Autodesk Fusion 360 part; units mm, degrees
(part 3 of 3)
sketch "Schizzo38" plane through (-271.3139, 0, 0) normal (-1, 0, 0) x (0, -1, 0)
  line L0 (10.9044, 16) -> (30.9044, 16)
  line L1 (30.9044, 16) -> (30.9044, 140)
  line L2 (19.4044, 140) -> (10.9044, 140)
  line L3 (10.9044, 140) -> (10.9044, 16)
  line L4 (19.4044, 140) -> (10.9044, 140) construction
  line L5 (10.9044, 140) -> (10.9044, 123.5) construction
  line L6 (10.9044, 123.5) -> (19.4044, 123.5) construction
  line L7 (19.4044, 123.5) -> (19.4044, 140) construction
  line L8 (28.9044, 123.5) -> (24.9044, 123.5)
  line L9 (24.9044, 123.5) -> (24.9044, 140)
  line L10 (24.9044, 140) -> (28.9044, 140)
  line L11 (28.9044, 140) -> (28.9044, 123.5)
  line L12 (26.9044, 123.5) -> (26.9044, 140) construction
  line L13 (19.4044, 123.5) -> (19.4044, 140)
  line L14 (30.9044, 140) -> (22.4044, 140)
  line L15 (22.4044, 140) -> (22.4044, 123.5)
  line L16 (22.4044, 123.5) -> (19.4044, 123.5)
  point P0 (10.9044, 140)
  dimension "d411" = 16.5
  dimension "d412" = 4
  dimension "d419" = 4
  constraint horizontal L4
  constraint vertical L5
  constraint horizontal L6
  constraint vertical L7
  constraint coincident L2.start L4.start
  constraint coincident P0 L2.end
  constraint horizontal L8
  constraint vertical L9
  constraint horizontal L10
  constraint vertical L11
  constraint coincident L4 L9.end
  constraint coincident L6 L8.start
  constraint midpoint L8 L12.start
  constraint midpoint L10 L12.end
  measures "d411" distance of L4 L6
  measures "d412" distance of L9 L11
  measures "d419" distance of L1 L12
extrude "Estrusione95" cut sketch "Schizzo38" against normal blind 5 contours L8 L9 L10 L11 L14 bodies 9
sketch "Schizzo28" plane through (0, -30.9044, 0) normal (0, -1, 0) x (1, 0, 0)
  line L0 (-261.8139, 0) -> (-253.3139, 0)
  line L1 (-253.3139, 0) -> (-253.3139, 16)
  line L2 (-255.3139, 16) -> (-255.3139, 140)
  line L3 (-255.3139, 140) -> (-271.3139, 140)
  line L4 (-271.3139, 140) -> (-271.3139, 16)
  line L5 (-273.3139, 16) -> (-273.3139, 0)
  line L6 (-273.3139, 0) -> (-273.3139, 16) construction
  line L7 (-273.3139, 0) -> (-253.3139, 0) construction
  line L8 (-261.8139, 0) -> (-253.3139, 0)
  line L9 (-253.3139, 0) -> (-253.3139, 16.5)
  line L10 (-261.8139, 20.1122) -> (-261.8139, 0)
  line L11 (-263.3139, 0) -> (-263.3139, 16.5) construction
  line L12 (-263.3139, 140) -> (-263.3139, 15) construction
  line L13 (-271.3139, 132) -> (-255.3139, 132) construction
  circle A0 centre (-263.3139, 132) radius 8
  circle A1 centre (-263.3139, 132) radius 4.1
  circle A2 centre (-263.3139, 132) radius 2
  line L14 (-261.8139, 16.5) -> (-261.8139, 0)
  line L15 (-273.3139, 0) -> (-264.8139, 0)
  line L16 (-264.8139, 0) -> (-264.8139, 16.5)
  line L17 (-264.8139, 16.5) -> (-261.8139, 16.5)
  line L18 (-261.8139, 16.5) -> (-261.8139, 0)
  line L19 (-261.8139, 0) -> (-253.3139, 0)
  line L20 (-253.3139, 0) -> (-253.3139, 16)
  line L21 (-253.3139, 16) -> (-255.3139, 16)
  line L22 (-255.3139, 16) -> (-255.3139, 140)
  line L23 (-271.3139, 140) -> (-271.3139, 16)
  line L24 (-271.3139, 16) -> (-273.3139, 16)
  line L25 (-273.3139, 16) -> (-273.3139, 0)
  line L26 (-273.3139, 0) -> (-264.8139, 0)
  line L27 (-264.8139, 0) -> (-264.8139, 16.5)
  line L28 (-264.8139, 16.5) -> (-261.8139, 16.5)
  line L29 (-273.3139, 16.5) -> (-253.3139, 16.5)
  line L30 (-253.3139, 16.5) -> (-253.3139, 0)
  line L31 (-253.3139, 0) -> (-273.3139, 0)
  line L32 (-273.3139, 0) -> (-273.3139, 16.5)
  line L33 (-255.3139, 140) -> (-271.3139, 140)
  line L34 (-263.3139, 136.1) -> (-271.3139, 136.1)
  line L35 (-271.3139, 136.1) -> (-271.3139, 127.9)
  line L36 (-271.3139, 127.9) -> (-263.3139, 127.9)
  line L37 (-263.3139, 127.9) -> (-263.3139, 136.1)
  point P0 (-271.3139, 0)
  dimension "d343" = 8
  dimension "d344" = 8.2
  dimension "d345" = 4
  dimension "d355" = 16.5
  constraint coincident L0.end L1.start
  constraint perpendicular L1 L7
  constraint horizontal L8
  constraint vertical L9
  constraint vertical L10
  constraint coincident L0.start L8.start
  constraint coincident L0.end L9
  constraint midpoint L7 L11.start
  constraint midpoint L3 L12.start
  constraint coincident L11 L12.end
  constraint coincident L4 L13.start
  constraint coincident L2 L13.end
  constraint perpendicular L12 L13
  constraint midpoint L13 A0.centre
  constraint tangent L3 A0
  constraint concentric A0 A1
  constraint concentric A0 A2
  constraint horizontal L29
  constraint vertical L30
  constraint horizontal L31
  constraint vertical L32
  constraint coincident L5.end L6.start
  constraint horizontal L34
  constraint vertical L35
  constraint horizontal L36
  constraint vertical L37
  constraint coincident A1 L34.start
  constraint coincident L12 L34.start
  constraint tangent A0 L35
  constraint tangent A1 L36
  measures "d343" distance of L3 L13.start
  measures "d344" diameter of A1
  measures "d345" diameter of A2
  measures "d355" distance of L29 P0
extrude "Estrusione80" cut sketch "Schizzo28" against normal blind 20 contours A2 L37 | A2 L37 bodies 9
extrude "Estrusione79" cut sketch "Schizzo28" against normal blind 1.5 contours A1 A2 L37 | A1 A2 L37 bodies 9
extrude "Estrusione81" cut sketch "Schizzo28" along normal blind 1 from surface at -20 contours A1 A2 L37 | A1 A2 L37 bodies 9
extrude "Estrusione122" cut sketch "Schizzo28" along normal blind 0.5 from surface at -20 contours L4 A0 L23 L35 L36 | A0 A1 L34 L36 | L4 A0 L23 L34 L35 picked at (-269.986, 131.5402) bodies 9
extrude "Estrusione82" cut sketch "Schizzo28" against normal blind 20 contours L2 L3 A0 L22 L33 | L3 L4 A0 L23 L33 L34 | L4 A0 L23 L34 L35 bodies 9
extrude "Estrusione77" cut sketch "Schizzo28" against normal blind 2 contours L0 L1 L2 L8 L9 L10 L14 L18 L19 L20 L21 L22 L29 L30 L31 | L4 L5 L15 L16 L23 L24 L25 L26 L27 L29 L31 L32 bodies 9
extrude "Estrusione78" cut sketch "Schizzo28" along normal blind 2 from surface at -20 contours L0 L1 L2 L8 L9 L10 L14 L18 L19 L20 L21 L22 L29 L30 L31 | L4 L5 L15 L16 L23 L24 L25 L26 L27 L29 L31 L32 bodies 9
sketch "Schizzo27" plane through (-273.3139, 0, 0) normal (-1, 0, 0) x (0, -1, 0)
  line L0 (12.9044, 0) -> (28.9044, 0)
  line L1 (28.9044, 16) -> (12.9044, 16)
  line L2 (12.9044, 16) -> (28.9044, 16) construction
  line L3 (28.9044, 16) -> (28.9044, 0) construction
  line L4 (28.9044, 0) -> (12.9044, 0) construction
  line L5 (12.9044, 0) -> (12.9044, 16) construction
  line L6 (20.9044, 16) -> (20.9044, 0) construction
  line L7 (12.9044, 8) -> (28.9044, 8)
  circle A0 centre (20.9044, 8) radius 8
  circle A1 centre (20.9044, 8) radius 2
  circle A2 centre (20.9044, 8) radius 4.1
  line L8 (12.9044, 16) -> (12.9044, 0)
  line L9 (28.9044, 0) -> (28.9044, 16)
  line L10 (20.9044, 12.1) -> (12.9044, 12.1)
  line L11 (12.9044, 12.1) -> (12.9044, 3.9)
  line L12 (12.9044, 3.9) -> (20.9044, 3.9)
  line L13 (20.9044, 3.9) -> (20.9044, 12.1)
  dimension "d317" = 4
  dimension "d322" = 8.2
  constraint horizontal L2
  constraint vertical L3
  constraint horizontal L4
  constraint vertical L5
  constraint coincident L0.end L3.end
  constraint coincident L1.end L2.start
  constraint midpoint L2 L6.start
  constraint midpoint L4 L6.end
  constraint midpoint L5 L7.start
  constraint midpoint L3 L7.end
  constraint midpoint L6 A0.centre
  constraint tangent L4 A0
  constraint concentric A0 A1
  constraint concentric A1 A2
  constraint horizontal L10
  constraint vertical L11
  constraint horizontal L12
  constraint vertical L13
  constraint coincident A2 L10.start
  constraint coincident L6 L10.start
  constraint tangent A2 L12
  constraint tangent A0 L11
  measures "d317" diameter of A1
  measures "d322" diameter of A2
extrude "Estrusione71" cut sketch "Schizzo27" against normal blind 20 contours L7 A1 L13 | L7 A1 L13 | L7 A1 L13 | L7 A1 L13 bodies 9
extrude "Estrusione72" cut sketch "Schizzo27" against normal blind 2 contours L1 A0 L9 | A0 L8 L10 L11 | L1 A0 L8 L10 bodies 9
extrude "Estrusione73" cut sketch "Schizzo27" against normal blind 20 contours L0 A0 L8 L12 | L0 A0 L9 | A0 L8 L11 L12 bodies 9
extrude "Estrusione74" cut sketch "Schizzo27" against normal blind 2 from surface at -18 contours L1 A0 L9 | A0 L8 L10 L11 | L1 A0 L8 L10 bodies 9
extrude "Estrusione75" cut sketch "Schizzo27" against normal blind 1 contours L7 A1 A2 L13 | L7 A1 A2 L13 | L7 A1 A2 L13 | L7 A1 A2 L13 bodies 9
extrude "Estrusione123" cut sketch "Schizzo27" against normal blind 0.5 contours L7 A0 A2 L12 | L7 A0 A2 L10 picked at (14.919, 5.0184) picked at (14.919, 10.9816) bodies 9
extrude "Estrusione76" cut sketch "Schizzo27" along normal blind 1.5 from surface at -20 contours L7 A1 A2 L13 | L7 A1 A2 L13 | L7 A1 A2 L13 | L7 A1 A2 L13 bodies 9
extrude "Estrusione105" add sketch "Schizzo1" along normal blind 16 separate body contours L191 L192 L193 L194 | L195 L196 L198 L199 | L196 L197 L198 L199 | A21 | A21 L202 L203 L204 L212 L213 L216 L217 | A21 L201 L202 L204 L207 L208 L220 L223 | L201 L202 L207 L208 L209 L210 | L202 L203 L212 L213 L214 L215 | L203 L204 L216 L217 L218 L219 | L201 L204 L220 L221 L222 L223 | A22 makes body 10
sketch "Schizzo41" plane through (0, -6.7942, 0) normal (0, -1, 0) x (1, 0, 0)
  line L0 (-212.9415, 0) -> (-192.9415, 0)
  line L1 (-192.9415, 0) -> (-192.9415, 16)
  line L2 (-192.9415, 16) -> (-212.9415, 16)
  line L3 (-212.9415, 16) -> (-212.9415, 0)
  line L4 (-212.9415, 16) -> (-192.9415, 16) construction
  line L5 (-192.9415, 16) -> (-192.9415, 0) construction
  line L6 (-192.9415, 0) -> (-212.9415, 0) construction
  line L7 (-212.9415, 0) -> (-212.9415, 16) construction
  line L8 (-202.9415, 16) -> (-202.9415, 0) construction
  line L9 (-212.9415, 8) -> (-192.9415, 8) construction
  line L10 (-201.4415, 16) -> (-204.4415, 16)
  line L11 (-204.4415, 16) -> (-204.4415, 0)
  line L12 (-204.4415, 0) -> (-201.4415, 0)
  line L13 (-201.4415, 0) -> (-201.4415, 16)
  line L14 (-201.4415, 16) -> (-204.4415, 0) construction
  line L15 (-204.4415, 16) -> (-201.4415, 0) construction
  line L16 (-212.9415, 0) -> (-192.9415, 0) construction
  line L17 (-192.9415, 16) -> (-195.9415, 16) construction
  line L18 (-195.9415, 16) -> (-195.9415, 13) construction
  line L19 (-195.9415, 13) -> (-192.9415, 13) construction
  line L20 (-192.9415, 13) -> (-192.9415, 16) construction
  line L21 (-193.9415, 15) -> (-197.9415, 15)
  line L22 (-197.9415, 15) -> (-197.9415, 11)
  line L23 (-197.9415, 11) -> (-193.9415, 11)
  line L24 (-193.9415, 11) -> (-193.9415, 15)
  line L25 (-193.9415, 15) -> (-197.9415, 11) construction
  line L26 (-197.9415, 15) -> (-193.9415, 11) construction
  line L27 (-197.9415, 15) -> (-193.9415, 15)
  line L28 (-193.9415, 15) -> (-193.9415, 16)
  line L29 (-193.9415, 16) -> (-197.9415, 16)
  line L30 (-197.9415, 16) -> (-197.9415, 15)
  point P0 (-192.9415, 0)
  point P1 (-202.9415, 8)
  point P2 (-195.9415, 13)
  dimension "d463" = 3
  dimension "d464" = 3
  dimension "d465" = 3
  dimension "d466" = 4
  dimension "d467" = 4
  constraint horizontal L4
  constraint vertical L5
  constraint horizontal L6
  constraint vertical L7
  constraint coincident P0 L0.end
  constraint coincident L2.end L3.start
  constraint midpoint L4 L8.start
  constraint midpoint L6 L8.end
  constraint midpoint L7 L9.start
  constraint midpoint L5 L9.end
  constraint horizontal L10
  constraint perpendicular L10 L11
  constraint parallel L10 L12
  constraint parallel L11 L13
  constraint coincident L14 P1
  constraint coincident L15 P1
  constraint midpoint L9 P1
  constraint collinear L12 L16
  constraint horizontal L17
  constraint vertical L18
  constraint horizontal L19
  constraint vertical L20
  constraint coincident L1.end L2.start
  constraint horizontal L21
  constraint perpendicular L21 L22
  constraint parallel L21 L23
  constraint parallel L22 L24
  constraint coincident L25 P2
  constraint coincident L26 P2
  constraint coincident P2 L18.end
  constraint horizontal L27
  constraint vertical L28
  constraint horizontal L29
  constraint vertical L30
  constraint coincident L17 L28.end
  constraint coincident L21.start L24.end
  measures "d463" distance of L11.end L12.end
  measures "d464" distance of L1.end L17.end
  measures "d465" distance of L1.end L19.end
  measures "d466" distance of L22.end L23.end
  measures "d467" distance of L21.end L22.end
extrude "Estrusione106" cut sketch "Schizzo41" against normal blind 50 contours L21 L22 L23 L24 L27 bodies 10
extrude "Estrusione107" cut sketch "Schizzo41" against normal blind 16.5 contours L2 L21 L27 L28 L29 L30 bodies 10
extrude "Estrusione108" cut sketch "Schizzo41" against normal blind 16.5 contours L0 L2 L10 L11 L12 L13 bodies 10
extrude "Estrusione109" cut sketch "Schizzo1" against normal blind 6 from surface at 16 contours L195 L196 L198 L199 bodies 10
extrude "Estrusione110" cut sketch "Schizzo1" against normal blind 10 from surface at 16 contours L196 L197 L198 L199 bodies 10
extrude "Estrusione111" cut sketch "Schizzo1" along normal blind 16 contours A22 bodies 10
extrude "Estrusione112" cut sketch "Schizzo1" against normal blind 6.4 from surface at 16 contours A21 bodies 10
extrude "Estrusione113" cut sketch "Schizzo1" along normal blind 5 contours A21 | A21 L202 L203 L204 L212 L213 L216 L217 | A21 L201 L202 L204 L207 L208 L220 L223 | L201 L202 L207 L208 L209 L210 | L202 L203 L212 L213 L214 L215 | L203 L204 L216 L217 L218 L219 | L201 L204 L220 L221 L222 L223 bodies 10
extrude "Estrusione114" cut sketch "Schizzo1" along normal blind 10 contours L201 L202 L207 L208 L209 L210 | L202 L203 L212 L213 L214 L215 | L203 L204 L216 L217 L218 L219 | L201 L204 L220 L221 L222 L223 bodies 10
sketch "Schizzo42" plane through (-192.9415, 0, 0) normal (1, 0, 0) x (0, 1, 0)
  line L0 (-6.7942, 0) -> (133.2058, 0)
  line L1 (133.2058, 0) -> (133.2058, 16)
  line L2 (133.2058, 16) -> (-6.7942, 16)
  line L3 (-6.7942, 16) -> (-6.7942, 0)
sketch "Schizzo43" plane through (-192.9415, 0, 0) normal (1, 0, 0) x (0, 1, 0)
  line L0 (-6.7942, 16) -> (133.2058, 16)
  line L1 (133.2058, 16) -> (133.2058, 0) construction
  line L2 (133.2058, 0) -> (-6.7942, 0)
  line L3 (-6.7942, 0) -> (-6.7942, 16)
  line L4 (-6.7942, 8) -> (133.2058, 8) construction
  circle A0 centre (1.2058, 8) radius 8
  circle A1 centre (1.2058, 8) radius 2
  circle A2 centre (1.2058, 8) radius 4.1
  line L5 (-2.8942, 16) -> (5.3058, 16)
  line L6 (5.3058, 16) -> (5.3058, 0)
  line L7 (5.3058, 0) -> (-2.8942, 0)
  line L8 (-2.8942, 0) -> (-2.8942, 16)
  line L9 (-2.8942, 16) -> (5.3058, 0) construction
  line L10 (5.3058, 16) -> (-2.8942, 0) construction
  point P0 (133.2058, 0)
  point P1 (-6.7942, 16)
  point P2 (2.7058, 8)
  point P3 (1.2058, 8)
  dimension "d502" = 4
  dimension "d504" = 8.2
  constraint horizontal L0
  constraint vertical L1
  constraint horizontal L2
  constraint vertical L3
  constraint coincident P0 L1.end
  constraint coincident L0.start L3.end
  constraint midpoint L3 L4.start
  constraint midpoint L1 L4.end
  constraint coincident L4 P3
  constraint tangent L2 A0
  constraint tangent L3 A0
  constraint concentric A0 A1
  constraint concentric A1 A2
  constraint horizontal L5
  constraint perpendicular L5 L6
  constraint parallel L5 L7
  constraint parallel L6 L8
  constraint coincident L9 P3
  constraint coincident L10 P3
  constraint coincident P3 A0.centre
  constraint tangent A2 L6
  constraint tangent A0 L7
  measures "d502" diameter of A1
  measures "d504" diameter of A2
extrude "Estrusione115" cut sketch "Schizzo43" against normal blind 20 contours L0 L3 A0 L8 | L0 A0 L5 L8 | L2 L3 A0 L8 | L2 A0 L7 L8 bodies 10
extrude "Estrusione116" cut sketch "Schizzo43" against normal blind 20 contours A1 bodies 10
extrude "Estrusione117" cut sketch "Schizzo43" against normal blind 1 contours A2 bodies 10
extrude "Estrusione118" cut sketch "Schizzo43" along normal blind 1 from surface at -20 contours A2 bodies 10
extrude "Estrusione119" cut sketch "Schizzo43" along normal blind 0.5 from surface at -20 contours L0 A0 L5 L8 | L0 A0 L5 L6 | A0 A2 L6 L8 picked at (0.746, 14.6721) bodies 10
extrude "Estrusione125" add sketch "Schizzo1" along normal blind 1 separate body contours L224 L227 L230 L231 L234 L243 L266 L268 | L224 L229 A23 L230 L231 L234 L243 L246 | L227 L228 L230 L231 L234 L245 L265 L266 L267 | L224 L229 A24 L232 L234 L247 L249 | L230 L231 L234 L243 L246 | L230 L231 L234 L243 L244 L267 | L227 L228 L230 L231 L233 L235 L257 L258 L260 | L234 L244 L266 L267 L268 | L234 L244 L265 L266 L267 | L224 L225 L232 L234 L247 L271 L272 | L229 A24 L234 L253 | L229 A23 L234 L253 | L230 L231 L234 L245 L246 | L230 L231 L234 L244 L245 L267 | L226 L227 L230 L231 L233 L237 L259 L260 | L228 A23 L234 L252 L253 | A23 L230 L231 L234 L245 L246 | L228 A23 L233 L251 L252 | A23 L230 L231 L233 L235 L236 | L232 L234 L247 L248 L270 | L232 L234 L247 L249 | A23 L234 | L228 A24 L234 L253 L254 | A24 L234 | L233 L238 L257 L258 L260 | L233 L238 L258 L259 L260 | A23 L233 | L226 L229 A23 L230 L231 L233 L236 L237 | L230 L231 L233 L235 L236 | L230 L231 L233 L235 L238 L258 | L225 L228 L232 L234 L250 L269 L270 L271 | L232 L234 L248 L250 L270 | L232 L234 L249 L250 | L234 L248 L270 L271 L272 | A24 L232 L234 L249 L250 | L230 L231 L233 L237 L238 L258 | L229 A23 L233 L251 | L230 L231 L233 L236 L237 | L225 L228 L232 L233 L239 L261 L262 L263 | L234 L248 L269 L270 L271 | L229 A24 L233 L251 | L228 A24 L233 L251 L254 | A24 L232 L233 L239 L240 | L226 L229 A24 L232 L233 L240 L242 | L225 L226 L232 L233 L242 L261 L264 | A24 L233 | L232 L233 L239 L241 L262 | L232 L233 L239 L240 | L233 L241 L261 L262 L264 | L233 L241 L261 L262 L263 | L232 L233 L240 L242 | L232 L233 L241 L242 L262 makes body 11
extrude "Estrusione124" add sketch "Schizzo1" along normal blind 83 contours L224 L227 L230 L231 L234 L243 L266 L268 | L224 L229 A23 L230 L231 L234 L243 L246 | L227 L228 L230 L231 L234 L245 L265 L266 L267 | L224 L229 A24 L232 L234 L247 L249 | L227 L228 L230 L231 L233 L235 L257 L258 L260 | L224 L225 L232 L234 L247 L271 L272 | L226 L227 L230 L231 L233 L237 L259 L260 | A23 L230 L231 L234 L245 L246 | A23 L230 L231 L233 L235 L236 | A23 L234 | A24 L234 | A23 L233 | L226 L229 A23 L230 L231 L233 L236 L237 | L225 L228 L232 L234 L250 L269 L270 L271 | A24 L232 L234 L249 L250 | L225 L228 L232 L233 L239 L261 L262 L263 | A24 L232 L233 L239 L240 | L226 L229 A24 L232 L233 L240 L242 | L225 L226 L232 L233 L242 L261 L264 | A24 L233 bodies 11
sketch "Schizzo44" plane through (0, 21.6443, 0) normal (0, -1, 0) x (1, 0, 0)
  line L0 (-605.2788, 0) -> (-528.2788, 0)
  line L1 (-528.2788, 0) -> (-528.2788, 83)
  line L2 (-528.2788, 83) -> (-605.2788, 83)
  line L3 (-605.2788, 83) -> (-605.2788, 0)
  circle A0 centre (-566.7788, 41.75) radius 11
  line L4 (-605.2788, 83) -> (-528.2788, 83) construction
  line L5 (-528.2788, 83) -> (-528.2788, 0) construction
  line L6 (-528.2788, 0) -> (-605.2788, 0) construction
  line L7 (-605.2788, 0) -> (-605.2788, 83) construction
  line L8 (-566.7788, 0) -> (-566.7788, 83) construction
  dimension "d543" = 22
  dimension "d544" = 41.25
  dimension "d546" = 77
  dimension "d547" = 83
  constraint horizontal L4
  constraint vertical L5
  constraint horizontal L6
  constraint vertical L7
  constraint coincident L0.end L1.start
  constraint coincident L2.end L3.start
  constraint midpoint L6 L8.start
  constraint midpoint L4 L8.end
  constraint coincident A0.centre L8
  measures "d543" diameter of A0
  measures "d544" distance of A0.centre L4
  measures "d546" distance of L5 L7
  measures "d547" distance of L4 L6
extrude "Estrusione126" cut sketch "Schizzo44" against normal blind 2 contours A0 bodies 11
extrude "Estrusione129" add sketch "Schizzo1" along normal blind 2 separate body contours L291 L292 L293 L294 makes body 12
extrude "Estrusione130" add sketch "Schizzo1" along normal blind 10 contours L304 L305 L306 L307 L309 | L313 L316 L317 L318 | L322 L323 L324 L325 | L326 L327 L328 L329 bodies 12
extrude "Estrusione131" add sketch "Schizzo1" along normal blind 2 separate body contours L343 L344 L345 L346 | L347 L348 L350 L355 | L348 L349 L350 L355 L356 | L348 L349 L353 L354 L355 L356 L358 L360 L363 L364 L365 L367 A25 | L355 L357 L358 L359 | L354 L355 L357 L358 L360 | L353 L356 L361 L363 L364 | L353 L361 L362 L363 | L353 L354 L365 L367 L368 A25 | L353 L366 L367 L368 | L365 L367 A25 | L365 L367 A25 | A26 makes body 13
extrude "Estrusione132" add sketch "Schizzo1" along normal blind 55 contours L343 L344 L345 L346 bodies 13
extrude "Estrusione133" add sketch "Schizzo1" along normal blind 100 from surface at 30 contours L347 L348 L350 L355 | L348 L349 L350 L355 L356 | L355 L357 L358 L359 | L354 L355 L357 L358 L360 | L353 L356 L361 L363 L364 | L353 L361 L362 L363 | L353 L354 L365 L367 L368 A25 | L353 L366 L367 L368 | L365 L367 A25 picked at (-531.8187, -95.3723) bodies 13
sketch "Schizzo46" plane through (0, -106.2441, 0) normal (0, -1, 0) x (1, 0, 0)
  line L0 (-605.2788, 0) -> (-528.2788, 0)
  line L1 (-528.2788, 0) -> (-528.2788, 55)
  line L2 (-528.2788, 55) -> (-605.2788, 55)
  line L3 (-605.2788, 55) -> (-605.2788, 0)
  line L4 (-605.2788, 55) -> (-528.2788, 55) construction
  line L5 (-528.2788, 55) -> (-528.2788, 0) construction
  line L6 (-528.2788, 0) -> (-605.2788, 0) construction
  line L7 (-605.2788, 0) -> (-605.2788, 55) construction
  circle A0 centre (-542.2788, 8) radius 5.05
  line L8 (-605.2788, 0) -> (-528.2788, 0)
  line L9 (-542.2788, 8) -> (-542.2788, 55) construction
  line L10 (-538.0288, 27) -> (-546.5288, 27)
  line L11 (-546.5288, 27) -> (-546.5288, 41)
  line L12 (-546.5288, 41) -> (-538.0288, 41)
  line L13 (-538.0288, 41) -> (-538.0288, 27)
  line L14 (-538.0288, 27) -> (-546.5288, 41) construction
  line L15 (-546.5288, 27) -> (-538.0288, 41) construction
  line L16 (-605.2788, 27.5) -> (-528.2788, 27.5) construction
  line L17 (-542.2788, 13.05) -> (-528.2788, 13.05) construction
  point P0 (-528.2788, 0)
  point P1 (-542.2788, 34)
  dimension "d600" = 10.1
  dimension "d607" = 8
  dimension "d608" = 14
  dimension "d617" = 8.5
  dimension "d618" = 14
  dimension "d619" = 6.5
  dimension "d620" = 14
  dimension "d621" = 13.95
  constraint horizontal L4
  constraint vertical L5
  constraint horizontal L6
  constraint vertical L7
  constraint coincident L2.end L3.start
  constraint coincident P0 L0.end
  constraint coincident A0.centre L9.start
  constraint coincident L2 L9.end
  constraint perpendicular L2 L9
  constraint horizontal L10
  constraint perpendicular L10 L11
  constraint parallel L10 L12
  constraint parallel L11 L13
  constraint coincident L14 P1
  constraint coincident L15 P1
  constraint coincident L9 P1
  constraint midpoint L7 L16.start
  constraint midpoint L5 L16.end
  constraint coincident A0 L17.start
  constraint coincident L9 L17.start
  constraint coincident L5 L17.end
  constraint tangent A0 L17
  measures "d600" diameter of A0
  measures "d607" distance of L6 A0.centre
  measures "d608" distance of L5 A0.centre
  measures "d617" distance of L11.end L12.end
  measures "d618" distance of L10.end L11.end
  measures "d619" distance of P1 L16
  measures "d620" distance of L4 L12
  measures "d621" distance of L10 L17
extrude "Estrusione134" cut sketch "Schizzo46" against normal blind 3 contours A0 bodies 13
extrude "Estrusione135" cut sketch "Schizzo1" along normal blind 2 contours L365 L367 A25 | L365 L367 A25 | A26 bodies 13
extrude "Estrusione136" cut sketch "Schizzo46" against normal blind 2 contours L10 L11 L12 L13 bodies 13
equation "BeamLenght = 140 mm"
equation "d2 = BeamLenght"
equation "d4 = BeamLock"
equation "BeamSlotDepth = 16.5 mm"
equation "d10 = -BeamSlotDepth"
equation "d12 = -BeamSlotDepth"
equation "d68 = d67"
equation "d70 = d69"
equation "d73 = -4 mm - JointLockDepth"
equation "d75 = BeamScrewHole"
equation "d76 = JointLockDepth"
equation "d79 = -JointLockDepth"
equation "d89 = CableBoreSize"
equation "d90 = CableBoreSize"
equation "d93 = CableBoreSize"
equation "d94 = CableBoreSize"
equation "d129 = BeamSlotDepth"
equation "CableBoreSize = 4 mm"
equation "d132 = CableBoreSize"
equation "d135 = BeamSlotDepth"
equation "d136 = CableBoreSize"
equation "d149 = CableBoreSize"
equation "d150 = CableBoreSize"
equation "d164 = -4 mm - JointLockDepth"
equation "d166 = 15.00 mm + 3 mm"
equation "d170 = d169"
equation "d173 = RotationJontDiameter / 2"
equation "d174 = d171"
equation "d175 = d172"
equation "d177 = CableBoreSize"
equation "d184 = RotationJontDiameter"
equation "RotationJontDiameter = 10 mm"
equation "d186 = RotationJontDiameter + 0.1 mm"
equation "d191 = ( 16 mm - RotationJontDiameter ) / 2"
equation "d198 = ( 28 / 2 ) * 1 mm - ( RotationJontDiameter / 2 )"
equation "d247 = 10 mm + 2 mm"
equation "d266 = RotationJontDiameter / 2 + 1 mm - 0.5 mm"
equation "d270 = RotationJontDiameter / 2 + 1 mm"
equation "d271 = RotationJontDiameter"
equation "d280 = d258"
equation "d288 = RotationJontDiameter"
equation "d308 = BeamLenght"
equation "d314 = BeamSlotDepth"
equation "d317 = BeamScrewHole"
equation "BeamScrewHole = 4 mm"
equation "BeamLock = 8.2 mm"
equation "d322 = BeamLock"
equation "d330 = -JointLockDepth"
equation "d344 = BeamLock"
equation "d345 = BeamScrewHole"
equation "d351 = JointLockDepth"
equation "d355 = BeamSlotDepth"
equation "JointLockDepth = 1 mm"
equation "d382 = 4 mm + JointLockDepth"
equation "d390 = BeamScrewHole"
equation "d391 = BeamScrewHole"
equation "d396 = BeamScrewHole"
equation "d397 = BeamScrewHole"
equation "d398 = BeamLenght"
equation "d407 = BeamScrewHole"
equation "d408 = BeamSlotDepth - 2 mm"
equation "d411 = BeamSlotDepth"
equation "d412 = BeamScrewHole"
equation "d416 = -BeamSlotDepth"
equation "d431 = 3 mm - 0.2 mm"
equation "d460 = BeamLenght"
equation "d466 = BeamScrewHole"
equation "d467 = BeamScrewHole"
equation "d470 = -BeamSlotDepth"
equation "d472 = -BeamSlotDepth"
equation "d502 = BeamScrewHole"
equation "d507 = -JointLockDepth"
equation "d510 = JointLockDepth"
equation "d513 = JointLockDepth - JointLockStep"
equation "JointLockStep = 0.5 mm" comment "This is the step before the joint lock sink"
equation "d517 = JointLockDepth - JointLockStep"
equation "d519 = -JointLockDepth + JointLockStep"
equation "d522 = JointLockDepth - JointLockStep"
equation "d525 = -JointLockDepth + JointLockStep"
equation "d535 = 4 mm + 0.1 mm"
equation "d536 = 6 mm + 0.2 mm"
equation "d537 = 1 mm - 0.1 mm"
equation "d538 = 6 mm - 0.1 mm"
equation "d544 = 41.75 mm - 0.5 mm"
equation "d551 = 10 mm + 0.2 mm"
equation "d553 = 6 mm - 0.3 mm"
equation "d584 = 8 mm + ( 28.50 / 2 ) * 1 mm"
equation "d596 = 56 mm - 1 mm"
named bodies: "Beam", "Joint", "Base Joint", "Base Cover", "Joint Holder New", "Joint Holder 2 New", "Dual Axis Beam", "Long Joint", "Camera Holder", "Lamp", "BatteryHolder", "BatteryCover", "ElectronicCover"
